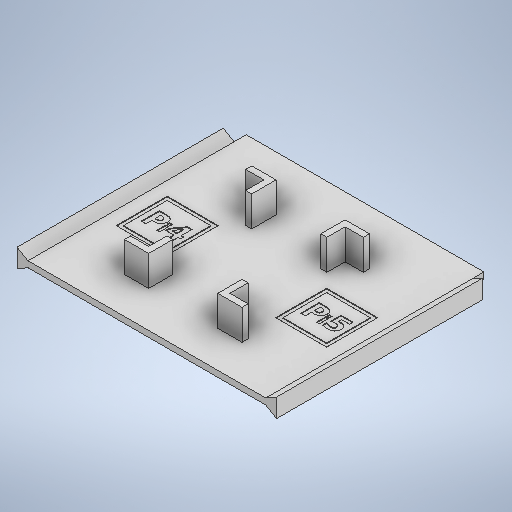
# Autodesk Inventor part: Suelo
Saved by Autodesk Inventor 2025.1 (Build 291241000, 241)
## iProperties
Created: 2025-11-20
Part Number: Suelo
Material: Genérico
Document SubType Name: Modeling
Designer: Diego
Density: 1 g/cm^3
Appearance: Valor por defecto
Author: Diego
Autodesk Inventor part; units mm, degrees
ref_plane "YZ Plane" through (0, 0, 0) normal (1, 0, 0) x (0, 1, 0)
ref_plane "XZ Plane" through (0, 0, 0) normal (0, 1, 0) x (-1, 0, 0)
ref_plane "XY Plane" through (0, 0, 0) normal (0, 0, 1) x (1, 0, 0)
sketch "Boceto1" plane through (0, 0, 0) normal (0, 0, 1) x (1, 0, 0)
  line L0 (-107.4375, 9.96) -> (-116.4375, 15.1562)
  line L1 (-116.4375, 15.1562) -> (-116.4375, -0.2361)
  line L2 (-116.4375, -0.2361) -> (-107.4375, 4.96)
  line L3 (-107.4375, 9.96) -> (-98.4042, 9.96) construction
  line L4 (-107.4375, 4.96) -> (-97.9616, 4.96) construction
  line L5 (-107.4375, 12.46) -> (-107.4375, 9.96) construction
  line L6 (-107.4375, 12.46) -> (-107.4375, 9.96) construction
  line L7 (-107.4375, 2.46) -> (-107.4375, 4.96) construction
  line L8 (88.5625, 12.46) -> (88.5625, 9.96) construction
  line L9 (88.5625, 12.46) -> (88.5625, 9.96) construction
  line L10 (97.5625, -0.2361) -> (88.5625, 4.96)
  line L11 (88.5625, 9.96) -> (97.5625, 15.1562)
  line L12 (97.5625, 15.1562) -> (97.5625, -0.2361)
  line L13 (88.5625, 4.96) -> (88.5625, 4.96) construction
  line L14 (88.5625, 4.96) -> (88.5625, 4.96) construction
  line L15 (88.5625, 4.96) -> (88.5625, 4.96)
  line L16 (88.5625, 7.46) -> (88.5625, 4.96)
  line L17 (88.5625, 4.96) -> (88.5625, 4.96)
  line L18 (88.5625, 9.96) -> (88.5625, 7.46)
  line L19 (-107.4375, 9.96) -> (-107.4375, 4.96)
  point P0 (0, 0)
  point P1 (-116.4375, 7.46)
  point P2 (97.5625, 7.46)
  point P3 (93.0625, 12.5581)
  point P4 (-111.9375, 12.5581)
  dimension "d0" = 60
  constraints: 40 end point, 5 vertical, 3 midpoint, 2 horizontal, 1 collinear, 1 parallel, 5 other
  measures "d0" angle of L0 L1
extrude "Extrusión1" add sketch "Boceto1" against normal blind 170
sketch "Boceto2" plane through (0, 0, 0) normal (0, 0, 1) x (1, 0, 0)
  line L0 (-107.4375, 9.96) -> (-107.4375, 4.96) projected
  line L1 (97.5625, -0.2361) -> (88.5625, 4.96) projected
  line L2 (-107.4375, 9.96) -> (88.5625, 9.96)
  line L3 (88.5625, 9.96) -> (88.5625, 4.96)
  line L4 (88.5625, 4.96) -> (-107.4375, 4.96)
  line L5 (-107.4375, 4.96) -> (-107.4375, 9.96)
  point P0 (0, 0)
  constraints: 8 end point, 2 parallel, 1 horizontal, 1 perpendicular
extrude "Extrusión2" add sketch "Boceto2" against normal blind 180
sketch "Boceto3" plane through (-107.4375, 9.96, 0) normal (0, 1, 0) x (1, 0, 0)
  line L0 (0, 0) -> (196, 0) projected
  line L1 (0, 0) -> (0, 170) projected
  line L2 (0, 180) -> (64.5, 180) construction
  line L3 (64.5, 180) -> (64.5, 35) construction
  line L4 (64.5, 35) -> (0, 35) construction
  line L5 (0, 35) -> (0, 180) construction
  line L6 (0, 180) -> (196, 180) projected
  line L7 (0, 170) -> (0, 180) projected
  line L8 (196, 180) -> (0, 180) construction
  line L9 (98, 180) -> (98, 0) construction
  line L10 (64.5, 82.5) -> (0, 82.5) construction
  line L11 (32.25, 180) -> (32.25, 35) construction
  line L12 (64.5, 100.5) -> (0, 100.5) construction
  line L13 (64.5, 64.5) -> (0, 64.5) construction
  line L14 (64.5, 35) -> (64.5, 50)
  line L15 (64.5, 50) -> (69.5, 50)
  line L16 (69.5, 50) -> (69.5, 30)
  line L17 (69.5, 30) -> (49.5, 30)
  line L18 (49.5, 30) -> (49.5, 35)
  line L19 (49.5, 35) -> (64.5, 35)
  line L20 (64.5, 130) -> (64.5, 115)
  line L21 (64.5, 115) -> (69.5, 115)
  line L22 (69.5, 115) -> (69.5, 135)
  line L23 (69.5, 135) -> (49.5, 135)
  line L24 (49.5, 135) -> (49.5, 130)
  line L25 (49.5, 130) -> (64.5, 130)
  line L26 (131.5, 35) -> (131.5, 50)
  line L27 (131.5, 50) -> (126.5, 50)
  line L28 (126.5, 50) -> (126.5, 30)
  line L29 (126.5, 30) -> (146.5, 30)
  line L30 (146.5, 30) -> (146.5, 35)
  line L31 (146.5, 35) -> (131.5, 35)
  line L32 (131.5, 115) -> (126.5, 115)
  line L33 (131.5, 130) -> (131.5, 115)
  line L34 (146.5, 130) -> (131.5, 130)
  line L35 (126.5, 115) -> (126.5, 135)
  line L36 (146.5, 135) -> (146.5, 130)
  line L37 (126.5, 135) -> (146.5, 135)
  point P0 (107.4375, 0)
  point P1 (32.25, 130)
  point P2 (131.5, 82.5)
  point P3 (131.5, 100.5)
  point P4 (131.5, 64.5)
  dimension "d14" = 36
  dimension "d21" = 30
  dimension "d22" = 5
  dimension "d23" = 20
  dimension "d24" = 5
  dimension "d25" = 64.5
  dimension "d26" = 20
  dimension "d27" = 47.5
  constraints: 66 end point, 22 symmetric about line, 10 point on line, 8 perpendicular, 4 midpoint, 2 horizontal, 2 parallel, 1 other
  measures "d14" distance between parallel lines of L13 L12
  measures "d21" distance between parallel lines of L0 L17
  measures "d22" distance of L17.end L18.end
  measures "d23" distance of L16.end L17.end
  measures "d24" distance of L14.end L15.end
  measures "d25" distance between parallel lines of L1 L14
  measures "d26" distance of L15.end L16.end
  measures "d27" distance between parallel lines of L19 L10
sketch "Boceto4" plane through (-107.4375, 9.96, 0) normal (0, 1, 0) x (1, 0, 0)
  line L0 (12.9564, 109.5347) -> (51.5436, 109.5347) construction
  line L1 (51.5436, 109.5347) -> (51.5436, 55.4653) construction
  line L2 (51.5436, 55.4653) -> (12.9564, 55.4653) construction
  line L3 (12.9564, 55.4653) -> (12.9564, 109.5347) construction
  line L4 (64.5, 100.5) -> (0, 100.5) construction
  line L5 (64.5, 82.5) -> (0, 82.5) construction
  line L6 (64.5, 64.5) -> (0, 64.5) construction
  line L7 (64.5, 180) -> (64.5, 35) construction
  line L8 (32.25, 180) -> (32.25, 35) construction
  line L9 (98, 180) -> (98, 0) construction
  line L10 (131.5, 100.5) -> (196, 100.5) construction
  line L11 (131.5, 82.5) -> (196, 82.5) construction
  line L12 (131.5, 64.5) -> (196, 64.5) construction
  line L13 (163.75, 180) -> (163.75, 35) construction
  line L14 (149.758, 112.112) -> (177.742, 112.112) construction
  line L15 (177.742, 112.112) -> (177.742, 52.888) construction
  line L16 (177.742, 52.888) -> (149.758, 52.888) construction
  line L17 (149.758, 52.888) -> (149.758, 112.112) construction
  line L18 (131.5, 180) -> (131.5, 35) construction
  line L19 (14.25, 64.5) -> (50.25, 64.5)
  line L20 (50.25, 64.5) -> (50.25, 100.5)
  line L21 (50.25, 100.5) -> (14.25, 100.5)
  line L22 (14.25, 100.5) -> (14.25, 64.5)
  line L23 (14.25, 64.5) -> (50.25, 100.5) construction
  line L24 (50.25, 64.5) -> (14.25, 100.5) construction
  line L25 (11.25, 61.5) -> (53.25, 61.5)
  line L26 (53.25, 61.5) -> (53.25, 103.5)
  line L27 (53.25, 103.5) -> (11.25, 103.5)
  line L28 (11.25, 103.5) -> (11.25, 61.5)
  line L29 (181.75, 64.5) -> (145.75, 64.5)
  line L30 (145.75, 64.5) -> (145.75, 100.5)
  line L31 (145.75, 100.5) -> (181.75, 100.5)
  line L32 (181.75, 100.5) -> (181.75, 64.5)
  line L33 (181.75, 64.5) -> (145.75, 100.5) construction
  line L34 (145.75, 64.5) -> (181.75, 100.5) construction
  line L35 (184.75, 61.5) -> (142.75, 61.5)
  line L36 (142.75, 61.5) -> (142.75, 103.5)
  line L37 (142.75, 103.5) -> (184.75, 103.5)
  line L38 (184.75, 103.5) -> (184.75, 61.5)
  spline S0 degree 2 poles (29.9202, 85.2897) (29.9202, 84.2443) (29.2516, 82.3481) (28.6317, 81.716) knots 0 0 0 1 2 2 2
  spline S1 degree 2 poles (28.6317, 81.716) (28.2549, 81.3148) (27.331, 80.6584) (26.784, 80.4275) knots 0 0 0 1 2 2 2
  spline S2 degree 2 poles (26.784, 80.4275) (26.2249, 80.1965) (24.9242, 79.9291) (24.122, 79.9291) knots 0 0 0 1 2 2 2
  line L39 (24.122, 79.9291) -> (22.1528, 79.9291)
  line L40 (22.1528, 79.9291) -> (22.1528, 75.0182)
  line L41 (22.1528, 75.0182) -> (18.3845, 75.0182)
  line L42 (18.3845, 75.0182) -> (18.3845, 90.0182)
  line L43 (18.3845, 90.0182) -> (24.2071, 90.0182)
  spline S3 degree 2 poles (24.2071, 90.0182) (25.4955, 90.0182) (27.3797, 89.5442) (28.1455, 89.0336) knots 0 0 0 1 2 2 2
  spline S4 degree 2 poles (28.1455, 89.0336) (28.9964, 88.4623) (29.9202, 86.5904) (29.9202, 85.2897) knots 0 0 0 1 2 2 2
  spline S5 degree 2 poles (26.0547, 85.1925) (26.0547, 85.8367) (25.4469, 86.7484) (25.0336, 86.9186) knots 0 0 0 1 2 2 2
  spline S6 degree 2 poles (25.0336, 86.9186) (24.4988, 87.1495) (23.5263, 87.2224) (22.6876, 87.2224) knots 0 0 0 1 2 2 2
  line L44 (22.6876, 87.2224) -> (22.1528, 87.2224)
  line L45 (22.1528, 87.2224) -> (22.1528, 82.7249)
  line L46 (22.1528, 82.7249) -> (22.4202, 82.7249)
  spline S7 degree 2 poles (22.4202, 82.7249) (22.9429, 82.7249) (23.891, 82.7492) (24.2435, 82.81) knots 0 0 0 1 2 2 2
  spline S8 degree 2 poles (24.2435, 82.81) (24.5474, 82.8586) (25.216, 83.1503) (25.3983, 83.3327) knots 0 0 0 1 2 2 2
  spline S9 degree 2 poles (25.3983, 83.3327) (25.7873, 83.6973) (26.0547, 84.5118) (26.0547, 85.1925) knots 0 0 0 1 2 2 2
  line L47 (33.6317, 75.0182) -> (31.2816, 75.0182)
  line L48 (31.2816, 75.0182) -> (31.2816, 82.5628)
  line L49 (31.2816, 82.5628) -> (33.6317, 82.5628)
  line L50 (33.6317, 82.5628) -> (33.6317, 75.0182)
  line L51 (33.7046, 83.6406) -> (31.2168, 83.6406)
  line L52 (31.2168, 83.6406) -> (31.2168, 85.472)
  line L53 (31.2168, 85.472) -> (33.7046, 85.472)
  line L54 (33.7046, 85.472) -> (33.7046, 83.6406)
  line L55 (47.2581, 78.519) -> (45.2281, 78.519)
  line L56 (45.2281, 78.519) -> (45.2281, 74.9818)
  line L57 (45.2281, 74.9818) -> (41.5936, 74.9818)
  line L58 (41.5936, 74.9818) -> (41.5936, 78.519)
  line L59 (41.5936, 78.519) -> (34.981, 78.519)
  line L60 (34.981, 78.519) -> (34.981, 81.3148)
  line L61 (34.981, 81.3148) -> (41.472, 90.0182)
  line L62 (41.472, 90.0182) -> (45.2281, 90.0182)
  line L63 (45.2281, 90.0182) -> (45.2281, 81.2176)
  line L64 (45.2281, 81.2176) -> (47.2581, 81.2176)
  line L65 (47.2581, 81.2176) -> (47.2581, 78.519)
  line L66 (41.5936, 81.2176) -> (41.5936, 86.3229)
  line L67 (41.5936, 86.3229) -> (37.7889, 81.2176)
  line L68 (37.7889, 81.2176) -> (41.5936, 81.2176)
  spline S10 degree 2 poles (161.4202, 85.4295) (161.4202, 84.3841) (160.7516, 82.4878) (160.1317, 81.8558) knots 0 0 0 1 2 2 2
  spline S11 degree 2 poles (160.1317, 81.8558) (159.7549, 81.4546) (158.831, 80.7982) (158.284, 80.5673) knots 0 0 0 1 2 2 2
  spline S12 degree 2 poles (158.284, 80.5673) (157.7249, 80.3363) (156.4242, 80.0689) (155.622, 80.0689) knots 0 0 0 1 2 2 2
  line L69 (155.622, 80.0689) -> (153.6528, 80.0689)
  line L70 (153.6528, 80.0689) -> (153.6528, 75.158)
  line L71 (153.6528, 75.158) -> (149.8845, 75.158)
  line L72 (149.8845, 75.158) -> (149.8845, 90.158)
  line L73 (149.8845, 90.158) -> (155.7071, 90.158)
  spline S13 degree 2 poles (155.7071, 90.158) (156.9955, 90.158) (158.8797, 89.684) (159.6455, 89.1734) knots 0 0 0 1 2 2 2
  spline S14 degree 2 poles (159.6455, 89.1734) (160.4964, 88.6021) (161.4202, 86.7301) (161.4202, 85.4295) knots 0 0 0 1 2 2 2
  spline S15 degree 2 poles (157.5547, 85.3323) (157.5547, 85.9765) (156.9469, 86.8882) (156.5336, 87.0583) knots 0 0 0 1 2 2 2
  spline S16 degree 2 poles (156.5336, 87.0583) (155.9988, 87.2893) (155.0263, 87.3622) (154.1876, 87.3622) knots 0 0 0 1 2 2 2
  line L74 (154.1876, 87.3622) -> (153.6528, 87.3622)
  line L75 (153.6528, 87.3622) -> (153.6528, 82.8647)
  line L76 (153.6528, 82.8647) -> (153.9202, 82.8647)
  spline S17 degree 2 poles (153.9202, 82.8647) (154.4429, 82.8647) (155.391, 82.889) (155.7435, 82.9498) knots 0 0 0 1 2 2 2
  spline S18 degree 2 poles (155.7435, 82.9498) (156.0474, 82.9984) (156.716, 83.2901) (156.8983, 83.4724) knots 0 0 0 1 2 2 2
  spline S19 degree 2 poles (156.8983, 83.4724) (157.2873, 83.8371) (157.5547, 84.6515) (157.5547, 85.3323) knots 0 0 0 1 2 2 2
  line L77 (165.1317, 75.158) -> (162.7816, 75.158)
  line L78 (162.7816, 75.158) -> (162.7816, 82.7026)
  line L79 (162.7816, 82.7026) -> (165.1317, 82.7026)
  line L80 (165.1317, 82.7026) -> (165.1317, 75.158)
  line L81 (165.2046, 83.7804) -> (162.7168, 83.7804)
  line L82 (162.7168, 83.7804) -> (162.7168, 85.6118)
  line L83 (162.7168, 85.6118) -> (165.2046, 85.6118)
  line L84 (165.2046, 85.6118) -> (165.2046, 83.7804)
  spline S20 degree 2 poles (178.2354, 80.2391) (178.2354, 79.06) (177.4331, 77.0665) (176.643, 76.3493) knots 0 0 0 1 2 2 2
  spline S21 degree 2 poles (176.643, 76.3493) (175.8529, 75.6321) (173.6892, 74.842) (172.109, 74.842) knots 0 0 0 1 2 2 2
  spline S22 degree 2 poles (172.109, 74.842) (170.4315, 74.8541) (168.0247, 75.4011) (167.2346, 75.7536) knots 0 0 0 1 2 2 2
  line L85 (167.2346, 75.7536) -> (167.2346, 79.0235)
  line L86 (167.2346, 79.0235) -> (167.575, 79.0235)
  spline S23 degree 2 poles (167.575, 79.0235) (167.8667, 78.8655) (168.5717, 78.4522) (169.143, 78.2334) knots 0 0 0 1 2 2 2
  spline S24 degree 2 poles (169.143, 78.2334) (169.6779, 78.0267) (170.784, 77.7472) (171.4526, 77.7472) knots 0 0 0 1 2 2 2
  spline S25 degree 2 poles (171.4526, 77.7472) (172.0361, 77.7472) (173.3975, 78.0389) (173.8108, 78.4279) knots 0 0 0 1 2 2 2
  spline S26 degree 2 poles (173.8108, 78.4279) (174.1147, 78.7318) (174.455, 79.4733) (174.455, 80.0932) knots 0 0 0 1 2 2 2
  spline S27 degree 2 poles (174.455, 80.0932) (174.455, 80.628) (174.0174, 81.3817) (173.6649, 81.6126) knots 0 0 0 1 2 2 2
  spline S28 degree 2 poles (173.6649, 81.6126) (173.1544, 81.953) (171.6957, 82.1475) (171.173, 82.1475) knots 0 0 0 1 2 2 2
  spline S29 degree 2 poles (171.173, 82.1475) (170.3464, 82.1475) (168.7784, 81.8801) (168.2071, 81.7342) knots 0 0 0 1 2 2 2
  line L87 (168.2071, 81.7342) -> (167.8788, 81.7342)
  line L88 (167.8788, 81.7342) -> (167.8788, 90.158)
  line L89 (167.8788, 90.158) -> (177.8221, 90.158)
  line L90 (177.8221, 90.158) -> (177.8221, 87.3258)
  line L91 (177.8221, 87.3258) -> (171.4404, 87.3258)
  line L92 (171.4404, 87.3258) -> (171.4404, 84.8339)
  spline S30 degree 2 poles (171.4404, 84.8339) (171.7443, 84.8582) (172.5831, 84.8825) (172.814, 84.8825) knots 0 0 0 1 2 2 2
  spline S31 degree 2 poles (172.814, 84.8825) (173.8959, 84.8825) (175.7192, 84.4449) (176.4364, 83.9951) knots 0 0 0 1 2 2 2
  spline S32 degree 2 poles (176.4364, 83.9951) (177.2873, 83.436) (178.2354, 81.5762) (178.2354, 80.2391) knots 0 0 0 1 2 2 2
  point P0 (107.4375, 0)
  point P1 (32.25, 82.5)
  point P2 (163.75, 82.5)
  dimension "d15" = 36
  dimension "d16" = 36
  dimension "d17" = 3
  constraints: 50 end point, 19 symmetric about line, 4 parallel, 3 midpoint, 2 perpendicular, 2 vertical, 1 horizontal, 1 point on line, 11 other
  measures "d15" distance of L21.end L20.end
  measures "d16" distance of L19.end L20.end
  measures "d17" distance between parallel lines of L22 L28
emboss "Repujado1" sketch "Boceto4" operation cut depth 0.6 direction (0, -1, 0)
extrude "Extrusión3" add sketch "Boceto3" along normal blind 25
equation "\"d3\" = L_base"
equation "\"d14\" = Font"
equation "\"d16\" = d15"
equation "\"L_base\" = 180"
equation "\"W_Pi\" = 64.5"
equation "\"L_Pi\" = 95"
equation "\"Font\" = 36"
